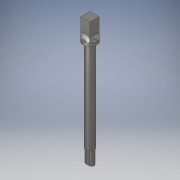
# Autodesk Inventor part: HOMBRO_EJE
Saved by Autodesk Inventor 2019 (Build 230136000, 136)
## iProperties
Created: 2020-02-12
Part Number: HOMBRO_EJE
Material: Acero, fundido1
Document SubType Name: Modeling
Designer: omar-
Density: 7.85 g/cm^3
Appearance: Semipulido
Author: omar-
Autodesk Inventor part; units mm, degrees
ref_plane "YZ Plane" through (0, 0, 0) normal (1, 0, 0) x (0, 1, 0)
ref_plane "XZ Plane" through (0, 0, 0) normal (0, 1, 0) x (-1, 0, 0)
ref_plane "XY Plane" through (0, 0, 0) normal (0, 0, 1) x (1, 0, 0)
sketch "Boceto1" plane through (0, 0, 0) normal (0, 1, 0) x (-1, 0, 0)
  circle A0 centre (0, 0) radius 2.75
  dimension "d0" = 5.5
  constraints: 1 centre point, 1 coincident
  measures "d0" diameter of A0
extrude "Extrusión1" add sketch "Boceto1" along normal blind 61
sketch "Boceto2" plane through (0, 61, 0) normal (0, 1, 0) x (1, 0, 0)
  circle A0 centre (0, 0) radius 4.5
  dimension "d3" = 9
  constraints: 1 centre point, 1 coincident
  measures "d3" diameter of A0
extrude "Extrusión2" add sketch "Boceto2" along normal blind 2
sketch "Boceto3" plane through (0, 63, 0) normal (0, 1, 0) x (1, 0, 0)
  line L0 (3, -3) -> (-3, -3)
  line L1 (-3, -3) -> (-3, 3)
  line L2 (-3, 3) -> (3, 3)
  line L3 (3, 3) -> (3, -3)
  line L4 (3, -3) -> (-3, 3) construction
  line L5 (-3, -3) -> (3, 3) construction
  point P0 (0, 0)
  dimension "d6" = 6
  dimension "d7" = 6
  constraints: 12 end point, 2 midpoint, 2 parallel, 1 horizontal, 1 perpendicular
  measures "d6" distance of L1.end L2.end
  measures "d7" distance of L0.end L1.end
extrude "Extrusión3" add sketch "Boceto3" along normal blind 12
fillet "Empalme1" radius 5.5 4 edges at (0, 63, 3) (3, 63, 0) (-3, 63, 0) (0, 63, -3)
sketch "Boceto4" plane through (0, 0, 0) normal (0, -1, 0) x (1, 0, 0)
  circle A0 centre (0, 0) radius 2.75 projected
  line L0 (-1.06, 0) -> (1.06, 0) construction
  line L1 (-1.06, 1.69) -> (1.06, 1.69)
  line L2 (1.06, -1.69) -> (-1.06, -1.69)
  arc A1 (-1.06, 1.69) -> (-1.06, -1.69) centre (-1.06, 0) ccw
  arc A2 (1.06, -1.69) -> (1.06, 1.69) centre (1.06, 0) ccw
  dimension "d14" = 5.5
  dimension "d15" = 1.69
  constraints: 8 end point, 4 point on circle, 4 tangent, 2 centre point, 1 horizontal, 1 midpoint, 1 parallel
  measures "d15" distance from line of L2 point (0, 0)
extrude "Extrusión4" add sketch "Boceto4" along normal blind 9 contours A2 L2 A1 L1
